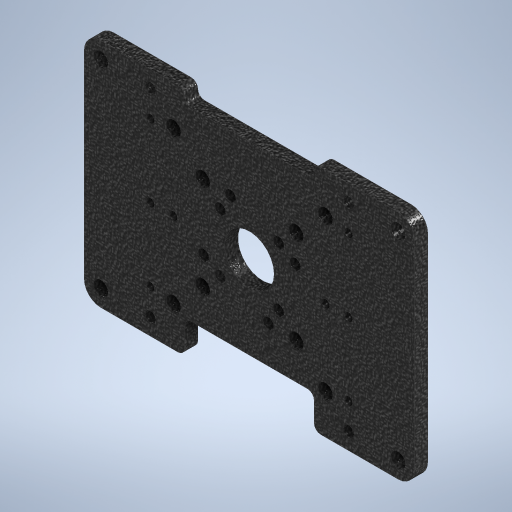
# Autodesk Inventor part: MotorMountLarge
Saved by Autodesk Inventor 2023 (Build 270158000, 158)
## iProperties
Created: 2023-11-23
Part Number: MotorMountLarge
Material: Generic
Document SubType Name: Modeling
Designer: aaron
Density: 1 g/cm^3
Appearance: Default
Author: aaron
Autodesk Inventor part; units mm, degrees
ref_plane "YZ Plane" through (0, 0, 0) normal (1, 0, 0) x (0, 1, 0)
ref_plane "XZ Plane" through (0, 0, 0) normal (0, 1, 0) x (-1, 0, 0)
ref_plane "XY Plane" through (0, 0, 0) normal (0, 0, 1) x (1, 0, 0)
sketch "Sketch1" plane through (0, 0, 0) normal (0, 0, 1) x (1, 0, 0)
  line L0 (-95, 70) -> (-5, 70)
  line L1 (0, 65) -> (0, 5)
  line L2 (-5, 0) -> (-95, 0)
  line L3 (-100, 5) -> (-100, 65)
  line L4 (-5, 65) -> (-95, 65)
  line L5 (-95, 65) -> (-95, 5)
  line L6 (-95, 5) -> (-5, 5)
  line L7 (-5, 5) -> (-5, 65)
  circle A0 centre (-50, 35) radius 7.5
  circle A1 centre (-50, 35) radius 12.5
  circle A2 centre (-50, 35) radius 15
  circle A3 centre (-50, 35) radius 20
  circle A4 centre (-50, 35) radius 32.5
  line L8 (-50, 35) -> (-50, -18.9163)
  line L9 (-50, 35) -> (-88.3245, -3.3245)
  circle A5 centre (-72.981, 12.019) radius 2.25
  circle A6 centre (-64.1421, 20.8579) radius 2.25
  circle A7 centre (-58.8388, 26.1612) radius 1.7
  line L10 (-50, 35) -> (-29.9707, -13.355)
  circle A8 centre (-44.2597, 21.1418) radius 1.7
  circle A9 centre (-41.1612, 26.1612) radius 1.7
  circle A10 centre (-35.8579, 20.8579) radius 2.25
  circle A11 centre (-27.019, 12.019) radius 2.25
  circle A12 centre (-36.1418, 40.7403) radius 1.7
  circle A13 centre (-41.1612, 43.8388) radius 1.7
  circle A14 centre (-35.8579, 49.1421) radius 2.25
  circle A15 centre (-27.019, 57.981) radius 2.25
  circle A16 centre (-55.7403, 48.8582) radius 1.7
  circle A17 centre (-58.8388, 43.8388) radius 1.7
  circle A18 centre (-64.1421, 49.1421) radius 2.25
  circle A19 centre (-72.981, 57.981) radius 2.25
  circle A20 centre (-63.8582, 29.2597) radius 1.7
  circle A21 centre (-95, 65) radius 2.25
  circle A22 centre (-5, 65) radius 2.25
  circle A23 centre (-5, 5) radius 2.25
  circle A24 centre (-95, 5) radius 2.25
  arc A25 (-95, 70) -> (-100, 65) centre (-95, 65) ccw
  arc A26 (0, 65) -> (-5, 70) centre (-5, 65) ccw
  arc A27 (-5, 0) -> (0, 5) centre (-5, 5) ccw
  arc A28 (-100, 5) -> (-95, 0) centre (-95, 5) ccw
  point P0 (0, 0)
  point P1 (0, 70)
  point P2 (-100, 0)
  point P3 (-37.5736, 5)
  point P4 (-37.5, 5)
  point P5 (-37.5628, 4.9739)
  dimension "d6" = 25
  dimension "d7" = 30
  dimension "d8" = 40
  dimension "d9" = 65
  dimension "d0" = 70
  dimension "d1" = 100
  dimension "d2" = 5
  dimension "d3" = 35
  dimension "d4" = 50
  dimension "d5" = 15
  dimension "d10" = 45
  dimension "d11" = 4.5
  dimension "d12" = 4.5
  dimension "d13" = 3.4
  dimension "d14" = 22.5
  dimension "d15" = 3.4
  dimension "d18" = 360
  dimension "d20" = 4.5
  dimension "d21" = 4.5
  dimension "d22" = 4.5
  dimension "d23" = 4.5
  dimension "d24" = 5
  constraints: 25 centre point, 22 end point, 10 point on line, 8 coincident, 8 point on circle, 8 tangent, 4 parallel, 3 equal radius, 2 perpendicular, 1 horizontal, 1 vertical, 48 other
  measures "d0" distance of point (0, 70) point (0, 0)
  measures "d1" distance of point (0, 0) point (-100, 0)
  measures "d2" distance between parallel lines of L0 L4
  measures "d3" distance from line of L0 A0.centre
  measures "d4" distance from line of L1 A0.centre
  measures "d5" diameter of A0
  measures "d10" angle of L8 L9
  measures "d11" diameter of A5
  measures "d12" diameter of A6
  measures "d13" diameter of A7
  measures "d14" angle of L8 L10
  measures "d15" diameter of A8
  measures "d20" diameter of A21
  measures "d21" diameter of A22
  measures "d22" diameter of A23
  measures "d23" diameter of A24
  measures "d24" radius of A25
extrude "Extrusion1" add sketch "Sketch1" along normal blind 4 contours L0 A26 L1 A27 L2 L10 A4 L6 A23 L7 A22 L4 A21 L5 A24 L9 A28 L3 A25 | L9 L6 A4 L8 L2 | L2 L8 A4 L10 | L9 A5 A4 L6 | L6 A24 L5 A21 L4 A4 A19 A5 L9 | A4 L8 L6 L10 | A4 L6 L8 | A4 A5 L9 A6 A3 L8 L6 | A4 A11 A15 L4 A22 L7 A23 L6 | L6 L10 A3 A10 A14 A18 A6 L9 A5 A4 A19 L4 A15 A11 | L6 L8 A3 L10 | L10 A8 A2 A12 A16 A20 L9 A6 A3 A18 A14 A10 | A3 L8 A2 A8 L10 | A3 A6 L9 A2 L8 | L8 A1 L10 A8 A2 | A2 L9 A7 A1 L8 | A2 A20 A16 A12 A8 L10 A1 A9 A13 A17 A7 L9 | L8 A0 L10 A1 | A1 A7 L9 A0 L8 | A4 L4 | L10 A0 L9 A7 A1 A17 A13 A9
sketch "Sketch2" plane through (0, 0, 4) normal (0, 0, 1) x (1, 0, 0)
  circle A0 centre (-50, 35) radius 7.5 projected
  line L0 (-50, 35) -> (3.4724, 35)
  line L1 (-20, 76.2111) -> (-20, -31.3319)
  line L2 (0, 5) -> (0, 65) projected
  line L3 (-26.988, 80.2967) -> (-26.988, -17.3618)
  line L4 (-50, 35) -> (-50, 0)
  line L5 (10.7091, 10) -> (-109.8814, 10)
  line L6 (9.3912, 66) -> (-107.2455, 66)
  line L7 (-5, 70) -> (-95, 70) projected
  line L8 (-95, 0) -> (-5, 0) projected
  line L9 (-30.4, 76.2111) -> (-30.4, 0)
  line L10 (-50, 0) -> (-30.4, 0)
  circle A1 centre (-26.988, 35) radius 1.25
  circle A2 centre (-20, 35) radius 1.25
  line L11 (-107.2455, 5) -> (19.174, 5)
  line L12 (8.4473, 65) -> (-108.1237, 65)
  line L13 (-105.6062, 57) -> (15.7808, 57)
  line L14 (8.4473, 13) -> (-108.1237, 13)
  circle A3 centre (-20, 65) radius 1.65
  circle A4 centre (-20, 5) radius 1.65
  circle A5 centre (-20, 57) radius 1.25
  circle A6 centre (-20, 13) radius 1.25
  circle A7 centre (-73.012, 35) radius 1.25
  circle A8 centre (-80, 35) radius 1.25
  circle A9 centre (-80, 65) radius 1.65
  circle A10 centre (-80, 5) radius 1.65
  circle A11 centre (-80, 57) radius 1.25
  circle A12 centre (-80, 13) radius 1.25
  line L15 (-5, 0) -> (-95, 0)
  line L16 (-69.6, 76.2111) -> (-69.6, 0)
  line L17 (-69.6, 70) -> (-30.4, 70)
  point P0 (0, 0)
  point P1 (-69.6, 66)
  point P2 (-30.4, 66)
  point P3 (-30.4, 10)
  point P4 (-69.6, 10)
  dimension "d27" = 20
  dimension "d28" = 26.988
  dimension "d29" = 4
  dimension "d30" = 10
  dimension "d31" = 30.4
  dimension "d32" = 2.5
  dimension "d33" = 2.5
  dimension "d34" = 5
  dimension "d35" = 5
  dimension "d36" = 13
  dimension "d37" = 13
  dimension "d38" = 3.3
  dimension "d39" = 3.3
  dimension "d40" = 2.5
  dimension "d41" = 2.5
  constraints: 30 end point, 16 point on line, 12 centre point, 10 symmetric about line, 7 horizontal, 4 vertical, 1 midpoint, 6 other
  measures "d27" distance between parallel lines of L1 L2
  measures "d28" distance between parallel lines of L2 L3
  measures "d29" distance between parallel lines of L6 L7
  measures "d30" distance between parallel lines of L5 L8
  measures "d31" distance between parallel lines of L2 L9
  measures "d32" diameter of A1
  measures "d33" diameter of A2
  measures "d34" distance between parallel lines of L8 L11
  measures "d35" distance between parallel lines of L7 L12
  measures "d36" distance between parallel lines of L8 L14
  measures "d37" distance between parallel lines of L13 L7
  measures "d38" diameter of A3
  measures "d39" diameter of A4
  measures "d40" diameter of A5
  measures "d41" diameter of A6
extrude "Extrusion2" cut sketch "Sketch2" against normal through all contours A1 L3 L0 | L0 L3 A1 | L5 L9 L11 L4 | L4 L11 L16 L5 | L3 A1 L0 | L0 A1 L3 | L11 L9 L8 L4 | L4 L8 L16 L11 | L6 L16 L7 L9 | A5 L1 L13 | L13 L1 A5 | A6 L1 L14 | L14 L1 A6 | A2 L1 L0 | L0 L1 A2 | A3 L6 L1 L12 | L12 L1 A3 | A9 L12 | L12 A9 L6 | L13 A5 L1 | L1 A5 L13 | L14 A6 L1 | L1 A6 L14 | L1 A2 L0 | L0 A2 L1 | A3 L1 L6 | L6 A9 | L12 A3 L1 | L1 L6 A3 L12 | A4 L1 L11 | L11 L1 A4 | A4 L11 L1 | L1 A3 L6 | L11 A4 L1 | A10 L11 | L11 A10 | A11 L13 | L13 A11 | A12 L14 | L14 A12 | A7 | A8
fillet "Fillet1" radius 2 8 edges at (-69.6, 70, 2) (-69.6, 66, 2) (-30.4, 70, 2) (-30.4, 66, 2) (-30.4, 0, 2) (-30.4, 10, 2) (-69.6, 10, 2) (-69.6, 0, 2)
equation "\"d3\" = 0.5 * d0"
equation "\"d4\" = 0.5 * d1"
body "Solid1"
